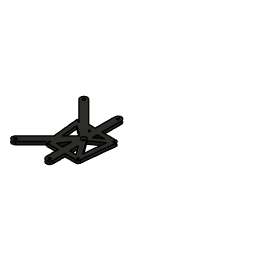
sensors-plate_lidar2d_ydlidar-x4_support (Autodesk Fusion 360 design; units mm, degrees)
Autodesk Fusion 360 part; units mm, degrees
note: some values were not read from the file. Chosen so that the rebuilt part matches the saved one: which face or edge a step refers to. Set by a fixed rule: which sketch regions a step uses.
sketch "Sketch1" plane through (0, 392, 0) normal (0, 1, 0) x (-1, 0, 0)
  circle A0 centre (120, -60) radius 2
  circle A1 centre (0, 120) radius 2
  circle A2 centre (120, 120) radius 2
  circle A3 centre (-120, 0) radius 2
  circle A4 centre (0, -120) radius 2
  circle A5 centre (0, -60) radius 2
  circle A6 centre (165.5, 26.5835) radius 2.5
  circle A7 centre (0, 0) radius 2
  circle A8 centre (60, 120) radius 2
  circle A9 centre (-165.5, -26.5835) radius 2.5
  circle A10 centre (165.5, 78.1855) radius 2.5
  circle A11 centre (120, 0) radius 2
  circle A12 centre (120, -120) radius 2
  circle A13 centre (-60, 60) radius 2
  circle A14 centre (-60, 120) radius 2
  circle A15 centre (-120, -60) radius 2
  circle A16 centre (60, 60) radius 2
  circle A17 centre (0, 60) radius 2
  circle A18 centre (165.5, -26.5835) radius 2.5
  circle A19 centre (60, -60) radius 2
  circle A20 centre (-165.5, 26.5835) radius 2.5
  circle A21 centre (60, 0) radius 2
  circle A22 centre (120, 60) radius 2
  circle A23 centre (165.5, -78.1855) radius 2.5
  circle A24 centre (-120, 60) radius 2
  circle A25 centre (-120, 120) radius 2
  circle A26 centre (-60, -120) radius 2
  circle A27 centre (-165.5, 78.1855) radius 2.5
  circle A28 centre (-120, -120) radius 2
  circle A29 centre (-60, 0) radius 2
  circle A30 centre (60, -120) radius 2
  circle A31 centre (-165.5, -78.1855) radius 2.5
  circle A32 centre (-60, -60) radius 2
  line L0 (-176, 131) -> (-176, -131)
  line L1 (-176, -131) -> (176, -131)
  line L2 (176, -131) -> (176, 131)
  line L3 (176, 131) -> (-176, 131)
  circle A33 centre (-120, 60) radius 6
  circle A34 centre (-120, -60) radius 6
  circle A35 centre (-120, 0) radius 6
  circle A36 centre (-60, 60) radius 6
  circle A37 centre (-60, -60) radius 6
  line L4 (-126, -60) -> (-126, 60)
  line L5 (-114, -60) -> (-114, 60)
  line L6 (-124.2426, 4.2426) -> (-64.2426, 64.2426)
  line L7 (-115.7574, -4.2426) -> (-55.7574, 55.7574)
  line L8 (-64.2426, -64.2426) -> (-124.2426, -4.2426)
  line L9 (-115.7574, 4.2426) -> (-55.7574, -55.7574)
  line L10 (-120, 0) -> (120, 0) construction
  line L11 (-120, 120) -> (-120, -120) construction
  circle A38 centre (-145, 35) radius 1.4
  circle A39 centre (-95, 35) radius 1.4
  circle A40 centre (-151, -22) radius 1.4
  line L12 (-145, 35) -> (-95, 35) construction
  circle A41 centre (-89, -22) radius 1.4
  circle A42 centre (-145, 35) radius 4
  circle A43 centre (-151, -22) radius 4
  circle A44 centre (-89, -22) radius 4
  circle A45 centre (-95, 35) radius 4
  line L13 (-154.978, -21.5813) -> (-148.978, 35.4187)
  line L14 (-141.022, 34.5813) -> (-147.022, -22.4187)
  line L15 (-151, -18) -> (-89, -18)
  line L16 (-151, -26) -> (-89, -26)
  line L17 (-145, 39) -> (-95, 39)
  line L18 (-145, 31) -> (-95, 31)
  line L19 (-98.978, 34.5813) -> (-92.978, -22.4187)
  line L20 (-91.022, 35.4187) -> (-85.022, -21.5813)
  circle A46 centre (-120, 0) radius 4 construction
  line L21 (-148.2549, 32.675) -> (-123.2549, -2.325)
  line L22 (-141.7451, 37.325) -> (-116.7451, 2.325)
  line L23 (-153.315, -18.738) -> (-122.315, 3.262)
  line L24 (-148.685, -25.262) -> (-117.685, -3.262)
  line L25 (-98.2549, 37.325) -> (-123.2549, 2.325)
  line L26 (-91.7451, 32.675) -> (-116.7451, -2.325)
  line L27 (-91.315, -25.262) -> (-122.315, -3.262)
  line L28 (-86.685, -18.738) -> (-117.685, 3.262)
  circle A47 centre (-120, 60) radius 2.15
  circle A48 centre (-120, -60) radius 2.15
  circle A49 centre (-60, -60) radius 2.15
  circle A50 centre (-120, 0) radius 2.15
  circle A51 centre (-60, 60) radius 2.15
  dimension "d212" = 12
  dimension "d213" = 2.8
  dimension "d214" = 35
  dimension "d216" = 50
  dimension "d217" = 57
  dimension "d218" = 62
  dimension "d219" = 8
  dimension "d220" = 8
  dimension "d221" = 0.15
  dimension "d222" = 0.15
  dimension "d223" = 0.15
  dimension "d224" = 0.15
  dimension "d225" = 0.15
  constraint concentric A24 A33
  constraint concentric A15 A34
  constraint concentric A3 A35
  constraint concentric A13 A36
  constraint concentric A32 A37
  constraint equal A33 A35
  constraint equal A33 A36
  constraint equal A33 A34
  constraint equal A33 A37
  constraint coincident A34 L4.start
  constraint coincident A33 L4.end
  constraint coincident A34 L5.start
  constraint coincident A33 L5.end
  constraint coincident A35 L6.start
  constraint coincident A36 L6.end
  constraint coincident A35 L7.start
  constraint coincident A36 L7.end
  constraint coincident A37 L8.start
  constraint coincident A35 L8.end
  constraint coincident A35 L9.start
  constraint coincident A37 L9.end
  constraint tangent A33 L4
  constraint tangent A33 L5
  constraint tangent A36 L6
  constraint tangent A36 L7
  constraint tangent A34 L4
  constraint tangent A34 L5
  constraint tangent A37 L8
  constraint tangent A37 L9
  constraint tangent A35 L8
  constraint tangent A35 L9
  constraint tangent A35 L7
  constraint tangent A35 L6
  constraint coincident A3.centre A35.centre
  constraint coincident A11.centre L10.end
  constraint coincident A25.centre L11.start
  constraint coincident A28.centre L11.end
  constraint equal A38 A39
  constraint symmetric L11 A38 A39
  constraint coincident A38.centre L12.start
  constraint coincident A39.centre L12.end
  constraint symmetric L11 A40 A41
  constraint equal A38 A40
  constraint concentric A38 A42
  constraint concentric A40 A43
  constraint concentric A41 A44
  constraint concentric A39 A45
  constraint equal A42 A43
  constraint equal A42 A45
  constraint equal A42 A44
  constraint coincident A43 L13.start
  constraint coincident A42 L13.end
  constraint tangent A42 L13
  constraint coincident A42 L14.start
  constraint coincident A43 L14.end
  constraint tangent A42 L14
  constraint tangent A43 L13
  constraint tangent A43 L14
  constraint coincident A43 L15.start
  constraint coincident A44 L15.end
  constraint coincident A43 L16.start
  constraint coincident A44 L16.end
  constraint coincident A42 L17.start
  constraint coincident A45 L17.end
  constraint coincident A42 L18.start
  constraint coincident A45 L18.end
  constraint tangent A45 L17
  constraint tangent A42 L17
  constraint tangent A42 L18
  constraint tangent A45 L18
  constraint tangent A43 L15
  constraint tangent A43 L16
  constraint tangent A44 L15
  constraint tangent A44 L16
  constraint coincident A45 L19.start
  constraint coincident A44 L19.end
  constraint coincident A45 L20.start
  constraint coincident A44 L20.end
  constraint tangent A45 L19
  constraint tangent A45 L20
  constraint tangent A44 L19
  constraint tangent A44 L20
  constraint concentric A35 A46
  constraint coincident A42 L21.start
  constraint coincident A46 L21.end
  constraint tangent A46 L21
  constraint coincident A42 L22.start
  constraint coincident A46 L22.end
  constraint tangent A46 L22
  constraint coincident A43 L23.start
  constraint coincident A46 L23.end
  constraint tangent A46 L23
  constraint coincident A43 L24.start
  constraint coincident A46 L24.end
  constraint tangent A46 L24
  constraint tangent A42 L22
  constraint tangent A42 L21
  constraint tangent A43 L23
  constraint tangent A43 L24
  constraint coincident A45 L25.start
  constraint coincident A46 L25.end
  constraint tangent A46 L25
  constraint coincident A45 L26.start
  constraint coincident A46 L26.end
  constraint tangent A46 L26
  constraint coincident A44 L27.start
  constraint coincident A46 L27.end
  constraint tangent A46 L27
  constraint coincident A44 L28.start
  constraint coincident A46 L28.end
  constraint tangent A46 L28
  constraint tangent A45 L25
  constraint tangent A45 L26
  constraint tangent A44 L28
  constraint tangent A44 L27
  measures "d212" diameter of A33
  measures "d213" diameter of A38
  measures "d214" distance of L10 A38.centre
  measures "d216" distance of A38.centre A39.centre
  measures "d217" distance of A40.centre L12
  measures "d218" distance of A40.centre A41.centre
  measures "d219" diameter of A42
  measures "d220" diameter of A46
extrude "Extrude1" add sketch "Sketch1" along normal blind 5 contours A33 | A33 L4 L5 L17 | L5 A45 L17 L18 L25 | L4 L5 L17 L18 | L4 A42 L17 L18 L22 | L4 L5 L6 L18 L22 L25 | L6 A39 A45 | A42 | L5 L6 L18 L19 L25 | L5 L6 L25 | A45 L18 L19 L25 | L6 A39 A45 | A36 L6 L7 A45 L20 | A35 L4 L6 L21 L22 | L4 L14 L18 L21 L22 | A42 L14 L18 L22 | A42 A43 L13 L14 L21 L23 | L5 L6 L9 L19 L26 | A35 L5 L6 L9 L22 L25 | L6 L22 L25 | L6 A45 L18 L19 | L6 L18 L19 | A36 | L7 A45 L19 L20 L26 | A35 L4 L21 L23 | A35 L6 L22 L25 | A42 L14 L18 | A42 L14 L18 L21 | A43 | L5 L9 L26 | A35 L5 L9 L26 | L6 A45 L18 L19 L26 | A35 L22 L25 | L6 A45 L18 | L7 A44 L19 L20 L28 | A35 L4 L23 | L4 L14 L15 L23 L24 | A35 L21 L23 | A35 L21 L23 L25 | A43 L14 L15 L23 | L4 A43 L15 L16 L24 | L5 L7 L9 L26 L28 | A35 L5 L26 L28 | A35 L22 L26 L28 | L7 L9 L19 L26 | A35 L22 L23 L24 L25 L27 L28 | L9 A41 A44 | A35 L4 L8 L24 | A43 L14 L15 | A43 L14 L15 L24 | A34 L4 L5 L16 | L4 L5 L15 L16 | L5 L7 L28 | A35 L5 L28 | A35 L26 L28 | L7 L9 L28 | A44 L15 L19 L28 | L9 L15 L19 L28 | A35 L8 L24 | L4 L5 L8 L15 L24 | A34 | L5 L8 L15 L16 | A35 L5 L7 | L5 L7 L9 L15 L27 L28 | L9 L15 L19 | L9 A44 L15 L19 | L9 A41 A44 | A37 L8 L9 A44 L16 | A35 L24 L27 | A35 L5 L8 L24 L27 | L8 A44 L15 L16 L27 | A35 L5 L7 L27 | L9 A44 L15 L19 L27 | L9 A44 L19 | A37 | L5 L8 L15 L27
hole "Hole1" at (145, 392, 35) direction (0, 1, 0) diameter 2 depth 5 tip angle 180 countersink diameter 5.5 countersink angle 90
hole "Hole2" at (151, 392, -22) direction (0, 1, 0) diameter 2 depth 5 tip angle 180 countersink diameter 5.5 countersink angle 90
hole "Hole3" at (95, 392, 35) direction (0, 1, 0) diameter 2 depth 5 tip angle 180 countersink diameter 5.5 countersink angle 90
hole "Hole4" at (89, 392, -22) direction (0, 1, 0) diameter 2 depth 5 tip angle 180 countersink diameter 5.5 countersink angle 90
hole "Hole5" at (120, 397, 0) direction (0, -1, 0) diameter 4 depth 5 tip angle 180 countersink diameter 9 countersink angle 90
